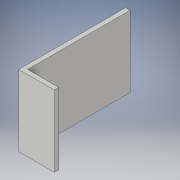
# Autodesk Inventor part: KillSwitchSupport
Saved by Autodesk Inventor 2017 (Build 210142000, 142)
## iProperties
Created: 2020-02-29
Part Number: KillSwitchSupport
Material: Generic
Document SubType Name: Modeling
Designer: S338674153
Density: 1 g/cm^3
Appearance: Default
Author: S338674153
Autodesk Inventor part; units mm, degrees
ref_plane "YZ Plane" through (0, 0, 0) normal (1, 0, 0) x (0, 1, 0)
ref_plane "XZ Plane" through (0, 0, 0) normal (0, 1, 0) x (-1, 0, 0)
ref_plane "XY Plane" through (0, 0, 0) normal (0, 0, 1) x (1, 0, 0)
sketch "Sketch2" plane through (0, 0, 0) normal (0, 1, 0) x (-1, 0, 0)
  line L0 (0, 0) -> (25.4, 0)
  line L1 (25.4, 0) -> (25.4, -3.175)
  line L2 (22.225, -3.175) -> (0, -3.175)
  line L3 (0, -3.175) -> (0, 0)
  line L4 (25.4, 0) -> (22.225, 0)
  line L5 (22.225, -3.175) -> (22.225, -76.2)
  line L6 (22.225, -76.2) -> (25.4, -76.2)
  line L7 (25.4, -76.2) -> (25.4, 0)
  dimension "d4" = 3.175
  dimension "d5" = 3.175
  dimension "d6" = 25.4
  dimension "d7" = 76.2
  constraints: 16 end point, 4 parallel, 2 horizontal, 2 perpendicular
  measures "d4" distance of L5.end L6.end
  measures "d5" distance of L2.end L0.start
  measures "d6" distance of L0.start L0.end
  measures "d7" distance of L6.end L0.end
extrude "Extrusion1" add sketch "Sketch2" along normal blind 50.8
body "Solid1"
